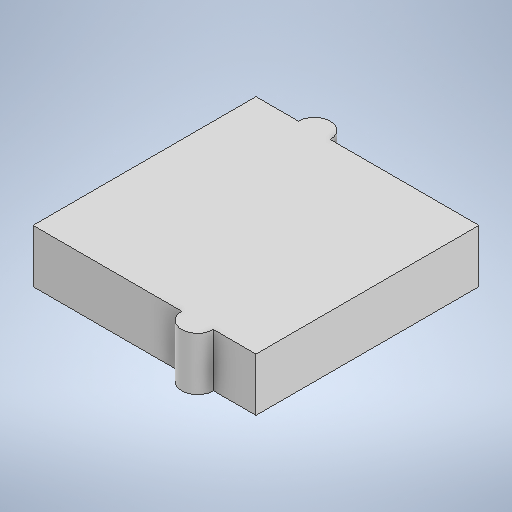
# Autodesk Inventor part: Kühler
Saved by Autodesk Inventor 2025.1 (Build 291241000, 241)
## iProperties
Created: 2025-01-26
Part Number: Kühler
Material: Generisch
Document SubType Name: Modeling
Designer: joebe
Density: 1 g/cm^3
Appearance: Vorgabe
Author: joebe
Autodesk Inventor part; units mm, degrees
ref_plane "YZ Plane" through (0, 0, 0) normal (1, 0, 0) x (0, 1, 0)
ref_plane "XZ Plane" through (0, 0, 0) normal (0, 1, 0) x (-1, 0, 0)
ref_plane "XY Plane" through (0, 0, 0) normal (0, 0, 1) x (1, 0, 0)
sketch "Skizze1" plane through (0, 0, 0) normal (0, 0, 1) x (1, 0, 0)
  line L0 (-10.5, 10.5) -> (10.5, 10.5)
  line L1 (10.5, 10.5) -> (10.5, -10.5)
  line L2 (10.5, -10.5) -> (-10.5, -10.5)
  line L3 (-10.5, -10.5) -> (-10.5, 10.5)
  line L4 (-10.5, 10.5) -> (10.5, -10.5) construction
  line L5 (10.5, 10.5) -> (-10.5, -10.5) construction
  point P0 (0, 0)
  dimension "d0" = 21
  dimension "d1" = 21
  constraints: 12 end point, 2 midpoint, 2 parallel, 1 horizontal, 1 perpendicular
  measures "d0" distance of L1.end L2.end
  measures "d1" distance of L0.end L1.end
extrude "Extrusion1" add sketch "Skizze1" along normal mid plane 5
sketch "Skizze2" plane through (0, 0, 2.5) normal (0, 0, 1) x (1, 0, 0)
  line L0 (10.5, 10.5) -> (-10.5, 10.5) projected
  circle A0 centre (-5, 10.5) radius 1.5
  circle A1 centre (5, -10.5) radius 1.5
  line L1 (-10.5, -10.5) -> (10.5, -10.5) projected
  point P0 (0, 0)
  point P1 (0, -10.5)
  point P2 (6.5, -10.5)
  point P3 (3.5, -10.5)
  point P4 (-6.5, 10.5)
  point P5 (-3.5, 10.5)
  dimension "d4" = 3
  dimension "d5" = 3
  dimension "d6" = 5
  dimension "d7" = 5
  constraints: 2 centre point, 1 horizontal alignment, 1 midpoint, 1 point on line
  measures "d4" diameter of A0
  measures "d5" diameter of A1
  measures "d6" horizontal distance of point (0, 0) A0.centre
  measures "d7" horizontal distance of point (0, 0) A1.centre
extrude "Extrusion2" add sketch "Skizze2" against normal blind 5 contours L0 A0 | A1 L1 picked at (-4.583, 11.1836) picked at (4.8227, -11.4322)
equation "\"d7\" = d6"
